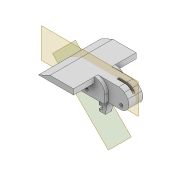
# Autodesk Inventor part: Middle_phalange
Saved by Autodesk Inventor 2022 (Build 260153000, 153)
## iProperties
Created: 2022-08-27
Part Number: Middle_phalange
Material: Generic
Document SubType Name: Modeling
Designer: dell
Density: 1 g/cm^3
Appearance: Default
Author: dell
Autodesk Inventor part; units mm, degrees
ref_plane "YZ Plane" through (0, 0, 0) normal (1, 0, 0) x (0, 1, 0)
ref_plane "XZ Plane" through (0, 0, 0) normal (0, 1, 0) x (-1, 0, 0)
ref_plane "XY Plane" through (0, 0, 0) normal (0, 0, 1) x (1, 0, 0)
sketch "Sketch1" plane through (0, 0, 0) normal (0, 0, 1) x (1, 0, 0)
  line L0 (0, 0) -> (-30, 0) construction
  line L1 (0, 14) -> (-30, 14)
  line L2 (-30, -14) -> (0, -14)
  arc A0 (0, -14) -> (0, 14) centre (0, 0) ccw
  arc A1 (-30, 14) -> (-30, -14) centre (-30, 0) ccw
  circle A2 centre (-30, 0) radius 1.55
  circle A3 centre (0, 0) radius 1.55
  line L3 (-30, 14) -> (0, 14)
  line L4 (0, 14) -> (0, 19)
  line L5 (0, 19) -> (-30, 19)
  line L6 (-30, 19) -> (-30, 14)
  line L7 (-43.4164, -4) -> (13.4164, -4)
  arc A4 (0, -14) -> (0, 14) centre (-7.746, 0) ccw
  line L8 (-30, 14) -> (-60, 14)
  arc A5 (-60, 14) -> (-30, -14) centre (21.7801, 71.5501) ccw
  point P0 (-15, 0)
  point P1 (7.746, -4)
  point P2 (-43.2985, -4.376)
  dimension "d0" = 28
  dimension "d1" = 30
  dimension "d2" = 3.1
  dimension "d3" = 3.1
  dimension "d7" = 5
  dimension "d13" = 4
  dimension "d27" = 16
  dimension "d48" = 100
  dimension "d49" = 0
  dimension "d50" = 30
  constraints: 20 end point, 10 point on circle, 6 centre point, 4 equal length, 4 tangent, 2 coincident, 2 horizontal, 1 midpoint, 1 perpendicular
  measures "d0" diameter of A1
  measures "d1" distance of L0.end L0.start
  measures "d2" diameter of A2
  measures "d3" diameter of A3
  measures "d7" distance of L4.end L1.start
  measures "d13" distance from line of L0.end L7
  measures "d27" radius of A4
  measures "d48" radius of A5
  measures "d49" distance between parallel lines of L1 L8
  measures "d50" distance of L1.end L8.end
extrude "Extrusion1" add sketch "Sketch1" along normal blind 20 contours A4 L7 A1 L1 | A1 A5 L8
sketch "Sketch3" plane through (0, 0, 0) normal (1, 0, 0) x (0, 1, 0)
  circle A0 centre (10, 10) radius 1
  point P0 (0, 0)
  dimension "d8" = 2
  dimension "d9" = 10
  dimension "d10" = 10
  constraints: 1 centre point
  measures "d8" diameter of A0
  measures "d9" horizontal distance of point (0, 0) A0.centre
  measures "d10" horizontal distance of point (0, 0) A0.centre
extrude "Extrusion2" cut sketch "Sketch3" along normal blind 200 and the other way blind 39
sketch "Sketch7" plane through (-30, 14, 0) normal (0, 1, 0) x (1, 0, 0)
  line L0 (17.45, -3.3) -> (62.8387, -3.3)
  line L1 (62.8387, -3.3) -> (62.8387, -16.7)
  line L2 (62.8387, -16.7) -> (17.45, -16.7)
  line L3 (17.45, -16.7) -> (17.45, -3.3)
  line L4 (30, -20) -> (-30, -20) projected
  line L5 (30, 0) -> (-30, 0) projected
  line L6 (31.55, -20) -> (28.45, -20) projected
  line L7 (31.55, 0) -> (28.45, 0) projected
  line L8 (17.45, 0) -> (41.8387, 0)
  line L9 (41.8387, 0) -> (41.8387, -20)
  line L10 (41.8387, -20) -> (17.45, -20)
  line L11 (17.45, -20) -> (17.45, 0)
  point P0 (17.45, -16.7)
  point P1 (30, -20)
  point P2 (31.55, -20)
  point P3 (41.8387, -16.7)
  point P4 (17.45, -3.3)
  point P5 (41.8387, -3.3)
  point P6 (31.55, 0)
  point P7 (30, 0)
  dimension "d37" = 3.3
  dimension "d38" = 3.3
  dimension "d39" = 11
  constraints: 16 end point, 4 parallel, 2 horizontal, 2 perpendicular, 1 collinear, 1 point on line
  measures "d37" distance between parallel lines of L4 L2
  measures "d38" distance between parallel lines of L5 L0
  measures "d39" distance from line of L7.end L3
extrude "Extrusion6" cut sketch "Sketch7" against normal blind 50 contours L11 L5 L7 L8 L9 L0 | L2 L9 L10 L6 L4 L11
sketch "Sketch8" plane through (0, 0, 0) normal (1, 0, 0) x (0, 1, 0)
  line L0 (14, 16.7) -> (-4, 16.7) projected
  line L1 (-4, 3.3) -> (-4, 16.7) projected
  line L2 (-4, 3.3) -> (14, 3.3) projected
  line L3 (14, 3.3) -> (14, 16.7) projected
  spline S0 degree 5 poles (11, 10) (11, 10.1494) (10.9722, 10.2982) (10.9163, 10.439) (10.8388, 10.5627) (10.6346, 10.7899) (10.5026, 10.887) (10.3537, 10.9562) (10.1942, 10.9944) (9.8787, 11.0043) (9.723, 10.9802) (9.5718, 10.9247) (9.4335, 10.8394) (9.1975, 10.6186) (9.1005, 10.4819) (9.0334, 10.3274) (9, 10.1636) (9, 9.7154) (9.0999, 9.4309) (9.3074, 9.1918) (9.5721, 9.0553) (10.0438, 8.9806) (10.2477, 9.0006) (10.4401, 9.0692) (10.6084, 9.1815) (10.8381, 9.4362) (10.9159, 9.5601) (10.9721, 9.7011) (11, 9.8502) (11, 10) knots 0 0 0 0 0 0 0.115733 0.115733 0.115733 0.115733 0.24846 0.24846 0.24846 0.24846 0.372945 0.372945 0.372945 0.372945 0.500007 0.500007 0.500007 0.500007 0.720991 0.720991 0.720991 0.720991 0.883979 0.883979 0.883979 0.883979 1 1 1 1 1 1 projected
  line L4 (14, 3.3) -> (14, 16.7) projected
  line L5 (10, 11) -> (14, 11)
  line L6 (14, 11) -> (14, 9)
  line L7 (14, 9) -> (10, 9)
  line L8 (10, 9) -> (10, 11)
  point P0 (0, 0)
  point P1 (10, 11)
  dimension "d42" = 2
  constraints: 8 end point, 2 parallel, 1 horizontal, 1 perpendicular, 1 point on line, 4 other
  measures "d42" distance between parallel lines of L5 L7
extrude "Extrusion7" cut sketch "Sketch8" along normal blind 10 and the other way blind 10 contours L3 L7 S0 L5
fillet "Fillet4" radius 2 2 edges at (-10, 10.6968, 9.2827) (-10, 10.6967, 10.7174)
fillet "Fillet5" radius 8 3 edges at (7.746, -4, 10) (0, 14, 13.85) (0, 14, 6.15)
fillet "Fillet6" radius 1 2 edges at (-12.55, -4, 18.35) (-12.55, -4, 1.65)
fillet "Fillet8" radius 10 2 edges at (-12.55, 14, 18.35) (-12.55, 14, 1.65)
ref_plane "Work Plane1" through (0, 0, 10) normal (0, 0, 1) x (1, 0, 0)
sketch "Sketch11" plane through (0, 0, 10) normal (0, 0, 1) x (1, 0, 0)
  arc A0 (6.1104, 8) -> (5.4828, 9) centre (-7.746, 0) ccw projected
  arc A1 (-0.8178, -4) -> (6.1104, 8) centre (-0.8178, 4) ccw projected
  line L0 (-0.8178, -4) -> (-43.4164, -4) projected
  arc A2 (-43.2985, -4.376) -> (-43.4164, -4) centre (-30, 0) ccw projected
  line L1 (-39, 9) -> (5.4828, 9) projected
  arc A3 (-12, 11) -> (-10, 13) centre (-12, 13) ccw projected
  line L2 (-12, 11) -> (-39, 11) projected
  line L3 (-60, 14) -> (-10, 14) projected
  line L4 (-10, 14) -> (-10, 13) projected
  circle A4 centre (-30, 0) radius 1.55 projected
  circle A5 centre (0, 0) radius 1.55 projected
  line L5 (-43.4164, -4) -> (-13.55, -4) projected
  line L6 (-16.3551, -4) -> (-19, -19)
  line L7 (-19, -19) -> (-25, -19)
  line L8 (-25, -19) -> (-25, -4)
  line L9 (-25, -17) -> (-22, -17)
  line L10 (-22, -17) -> (-22, -14)
  line L11 (-22, -14) -> (-25, -14)
  line L12 (-25, -14) -> (-25, -17)
  line L13 (-39, 11) -> (-39, 9) projected
  arc A6 (-60, 14) -> (-43.2985, -4.376) centre (21.7801, 71.5501) ccw projected
  point P0 (-25, -4)
  dimension "d77" = 15
  dimension "d78" = 25
  dimension "d79" = 80
  dimension "d80" = 2
  dimension "d82" = 3
  dimension "d84" = 3
  dimension "d85" = 6
  constraints: 14 end point, 3 parallel, 3 point on line, 2 perpendicular, 1 horizontal
  measures "d77" distance of L7.end L8.end
  measures "d78" distance from line of point (0, 0) L8
  measures "d79" angle of L5 L6
  measures "d80" distance between parallel lines of L7 L9
  measures "d82" distance of L9.end L10.end
  measures "d84" distance from line of L6.end L10
  measures "d85" distance from line of L6.end L8
extrude "Extrusion10" add sketch "Sketch11" along normal mid plane 6 contours A2 L8 L0 | L0 L6 L7 L8 L9 L10 L11 A2
ref_plane "Work Plane2" through (-43.4164, -4, 0) normal (-0.7071068, -0.7071068, 0) x (0, 0, 1)
sketch "Sketch13" plane through (-43.4164, -4, 0) normal (-0.7071068, -0.7071068, 0) x (0, 0, 1)
  line L0 (20, 0) -> (0, 0) projected
  line L1 (10, 39.4396) -> (10, -65.4576) projected
  circle A0 centre (10, 6.6802) radius 1
  line L2 (20, 17.0779) -> (20, 0) projected
  line L3 (0, 0) -> (0, 17.0779) projected
  line L4 (0, 17.0779) -> (20, 17.0779) projected
  point P0 (0, -27.8716)
  dimension "d90" = 2
  constraints: 1 centre point, 1 point on line
  measures "d90" diameter of A0
extrude "Extrusion12" cut sketch "Sketch13" along normal blind 10 and the other way blind 13.6 contours A0 L1 | L1 A0
sketch "Sketch14" plane through (0, 0, 20) normal (0, 0, 1) x (1, 0, 0)
  line L0 (-22.55, 14) -> (-60, 14) projected
  line L1 (-45, 14) -> (-56.1006, 8.8237)
  arc A0 (-60, 14) -> (-43.2985, -4.376) centre (21.7801, 71.5501) ccw projected
  point P0 (0, 0)
  dimension "d95" = 15
  dimension "d96" = 25
  constraints: 2 end point, 1 point on circle, 1 point on line
  measures "d95" distance of L0.end L1.start
  measures "d96" angle of L0 L1
extrude "Extrusion13" cut sketch "Sketch14" against normal blind 100
sketch "Sketch15" plane through (0, 0, 20) normal (0, 0, 1) x (1, 0, 0)
  line L0 (-45, 14) -> (-56.1006, 8.8237) projected
  line L1 (-22.55, 14) -> (-45, 14) projected
  arc A0 (-56.1006, 8.8237) -> (-43.2985, -4.376) centre (21.7801, 71.5501) ccw projected
  line L2 (-2.4545, 14) -> (-22.55, 14) projected
  line L3 (-56.1006, 8.8237) -> (-22.55, 8.8237)
  line L4 (-22.55, 8.8237) -> (-22.55, 14)
  point P0 (0, 0)
  constraints: 4 end point, 1 horizontal
extrude "Extrusion14" add sketch "Sketch15" along normal blind 20
mirror "Mirror1" about plane through (0, 0, 10) normal (0, 0, 1) of "Extrusion14"
body "Solid1"
